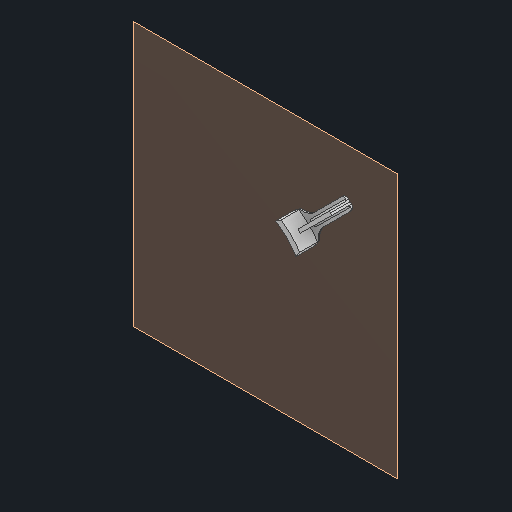
# Autodesk Inventor part: HourGuard
Saved by Autodesk Inventor 2023.1 (Build 271208000, 208)
## iProperties
Created: 2023-08-25
Part Number: HourGuard
Material: Generic
Document SubType Name: Modeling
Designer: washichi
Density: 1 g/cm^3
Appearance: Default
Author: washichi
Autodesk Inventor part; units mm, degrees
ref_plane "YZ Plane" through (0, 0, 0) normal (1, 0, 0) x (0, 1, 0)
ref_plane "XZ Plane" through (0, 0, 0) normal (0, 1, 0) x (-1, 0, 0)
ref_plane "XY Plane" through (0, 0, 0) normal (0, 0, 1) x (1, 0, 0)
ref_plane "Work Plane1" through (0, 0, 0) normal (0, 0, 1) x (1, 0, 0)
sketch "Sketch1" plane through (0, 0, 0) normal (0, 0, 1) x (1, 0, 0)
  circle A0 centre (0, 0) radius 78.5
  line L0 (0, 0) -> (103.944697, 103.944697)
  line L1 (0, 0) -> (147, 0) construction
  line L2 (103.944697, 103.944697) -> (102.17693, 105.712464)
  line L3 (103.944697, 103.944697) -> (105.679378, 102.270109)
  circle A1 centre (0, 0) radius 71
  line L4 (105.742236, 95.137281) -> (55.226256, 44.621302)
  line L5 (109.340638, 98.735683) -> (180.781021, 98.735683) construction
  line L6 (95.105862, 105.712464) -> (44.620391, 55.226993)
  line L7 (98.641396, 109.247998) -> (170.038634, 109.247998) construction
  line L8 (44.257728, 44.257728) -> (66.757728, 44.257728)
  line L9 (66.757728, 44.257728) -> (66.757728, 66.757728)
  line L10 (66.757728, 66.757728) -> (44.257728, 66.757728)
  line L11 (44.257728, 66.757728) -> (44.257728, 44.257728)
  line L12 (44.257728, 44.257728) -> (66.757728, 66.757728) construction
  line L13 (66.757728, 44.257728) -> (44.257728, 66.757728) construction
  arc A2 (102.17693, 105.712464) -> (95.105862, 105.712464) centre (98.641396, 102.17693) ccw
  arc A3 (105.742236, 95.137281) -> (105.679378, 102.270109) centre (102.206702, 98.672815) ccw
  line L14 (44.257728, 66.757728) -> (35.912715, 61.247669)
  line L15 (66.757728, 44.257728) -> (61.247669, 35.912715)
  point P0 (55.507728, 55.507728)
  point P1 (55.518047, 44.257728)
  point P2 (66.757728, 56.152774)
  point P3 (56.151126, 66.757728)
  point P4 (44.257728, 55.518047)
  dimension "d0" = 157
  dimension "d1" = 147
  dimension "d2" = 45
  dimension "d3" = 7.5
  dimension "d4" = 7.5
  dimension "d5" = 142
  dimension "d6" = 135
  dimension "d7" = 135
  dimension "d8" = 22.5
  dimension "d9" = 22.5
  dimension "d10" = 5
  dimension "d34" = 10
  dimension "d35" = 10
  constraints: 32 end point, 8 point on circle, 5 point on line, 4 centre point, 4 horizontal, 4 tangent, 3 equal length, 2 coincident, 2 midpoint, 2 parallel, 2 perpendicular, 1 equal radius
  measures "d0" diameter of A0
  measures "d1" distance of L0.start L0.end
  measures "d2" angle of L1 L0
  measures "d3" distance of L0.end L7.start
  measures "d4" distance of L0.end L5.start
  measures "d5" diameter of A1
  measures "d6" angle of L4 L5
  measures "d7" angle of L6 L7
  measures "d8" distance of L10.end L9.end
  measures "d9" distance of L9.end L8.end
  measures "d10" radius of A2
  measures "d34" distance of L10.end L14.end
  measures "d35" distance of L15.start L15.end
extrude "Extrusion1" add sketch "Sketch1" along normal blind 2 contours L15 A1 L8 A0 | A0 L8 L15 | L14 L11 A0 | A0 L11 A1 L14 | L8 A1 L4 A0 | A0 L4 L9 L8 | L11 L10 L6 A0 | A0 L6 A1 L11 | L4 A1 L0 A0 | A0 L0 L9 L4 | L9 L0 L3 A3 L4 | L6 L10 L0 A0 | A0 L0 A1 L6 | L6 A2 L2 L0 L10
sketch "Sketch2" plane through (0, 0, 2) normal (0, 0, 1) x (1, 0, 0)
  circle A0 centre (0, 0) radius 78.5
  circle A1 centre (0, 0) radius 71
  line L0 (105.679378, 102.270109) -> (103.944697, 103.944697)
  line L1 (103.944697, 103.944697) -> (61.51829, 61.51829)
  line L2 (103.944697, 103.944697) -> (163.944697, 103.944697) construction
  line L3 (103.944697, 103.944697) -> (102.17693, 105.712464)
  line L4 (44.257728, 66.757728) -> (44.257728, 55.518047)
  line L5 (55.518047, 44.257728) -> (66.757728, 44.257728)
  line L6 (46.257728, 66.757728) -> (46.257728, 55.518047)
  line L7 (55.518047, 46.257728) -> (66.757728, 46.257728)
  line L8 (61.51829, 61.51829) -> (60.113782, 62.942143)
  line L9 (60.113782, 62.942143) -> (62.922798, 60.094437)
  arc A2 (105.742236, 95.137281) -> (105.679378, 102.270109) centre (102.206702, 98.672815) ccw
  line L10 (62.922798, 60.094437) -> (105.679378, 102.270109)
  line L11 (60.113782, 62.942143) -> (102.530516, 105.358877)
  line L12 (60.113782, 62.942143) -> (120.100103, 62.942143) construction
  line L13 (46.257728, 55.518047) -> (46.257728, 53.862998)
  line L14 (55.518047, 46.257728) -> (53.862998, 46.257728)
  line L15 (56.151126, 66.757728) -> (44.257728, 66.757728)
  line L16 (44.257728, 66.757728) -> (35.912715, 61.247669)
  line L17 (66.757728, 44.257728) -> (61.247669, 35.912715)
  point P0 (58.399252, 46.257728)
  point P1 (63.422966, 46.257728)
  point P2 (46.257728, 63.422966)
  point P3 (46.257728, 58.399252)
  point P4 (44.257728, 64.834432)
  point P5 (64.834432, 44.257728)
  point P6 (65.800574, 42.808113)
  point P7 (42.808113, 65.800574)
  dimension "d13" = 157
  dimension "d14" = 7.5
  dimension "d16" = 135
  dimension "d21" = 2
  dimension "d22" = 2
  dimension "d25" = 60
  dimension "d26" = 2
  dimension "d27" = 4
  dimension "d28" = 45
  dimension "d32" = 10
  dimension "d33" = 10
  constraints: 26 end point, 4 point on circle, 3 horizontal, 2 centre point, 2 equal length, 2 parallel, 2 point on line, 1 coincident, 1 perpendicular, 1 vertical
  measures "d13" diameter of A0
  measures "d14" radial gap between concentric circles of A0 A1
  measures "d16" angle of L1 L2
  measures "d21" distance between parallel lines of L4 L6
  measures "d22" distance between parallel lines of L5 L7
  measures "d25" distance of L0.end L1.end
  measures "d26" distance of L1.end L8.end
  measures "d27" distance of L8.end L9.end
  measures "d28" angle of L12 L11
  measures "d32" distance of L4.start L16.end
  measures "d33" distance of L5.end L17.end
extrude "Extrusion2" add sketch "Sketch2" along normal blind 22 contours L17 A1 L5 A0 | A0 L4 A1 L16 | L5 A1 L14 L7 A0 | A0 L6 L13 A1 L4 | L7 L14 A1 L13 L6 A0 | L10 L9 L1 L0 | L1 L8 L11 L3
chamfer "Chamfer1" distance 2 angle 45 3 edges at (84.3011, 81.1823, 2) (81.3221, 84.1505, 2) (61.5183, 61.5183, 2)
chamfer "Chamfer2" distance 5 angle 45 3 edges at (66.7577, 56.1528, 1) (56.1511, 66.7577, 1) (61.5183, 61.5183, 24)
body "Solid1"
